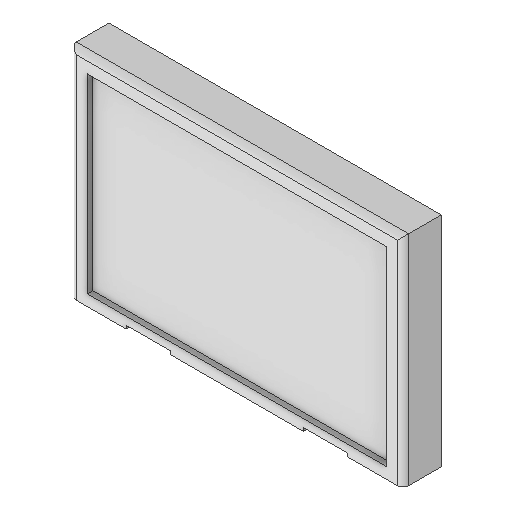
# Autodesk Inventor part: PLATE 2
Saved by Autodesk Inventor 2025.3 (Build 293356030, 356C)
## iProperties
Created: 2025-09-26
Part Number: PLATE 2
Material: 일반
Document SubType Name: Modeling
Designer: joseph
Density: 1 g/cm^3
Appearance: 기본값
Author: joseph
Autodesk Inventor part; units mm, degrees
ref_plane "YZ Plane" through (0, 0, 0) normal (1, 0, 0) x (0, 1, 0)
ref_plane "XZ Plane" through (0, 0, 0) normal (0, 1, 0) x (-1, 0, 0)
ref_plane "XY Plane" through (0, 0, 0) normal (0, 0, 1) x (1, 0, 0)
sketch "스케치1" plane through (0, 0, 0) normal (0, 0, 1) x (1, 0, 0)
  line L0 (150, 3) -> (-150, 3)
  line L1 (-150, 3) -> (-150, 200)
  line L2 (-150, 200) -> (150, 200)
  line L3 (150, 200) -> (150, 3)
  point P0 (0, 0)
  dimension "d0" = 300
  dimension "d1" = 197
  constraints: 8 end point, 2 parallel, 1 horizontal, 1 perpendicular
  measures "d0" distance of L1.end L2.end
  measures "d1" distance of L0.end L1.end
extrude "돌출1" add sketch "스케치1" along normal blind 34.5
fillet "모깎기1" radius 5 3 edges at (150, 101.5, 34.5) (-150, 101.5, 34.5) (0, 200, 34.5)
sketch "스케치2" plane through (0, 0, 0) normal (0, 0, -1) x (-1, 0, 0)
  line L0 (-150, 200) -> (150, 200) projected
  line L1 (-150, 3) -> (-150, 200) projected
  line L2 (150, 3) -> (-150, 3) projected
  line L3 (150, 200) -> (150, 3) projected
  line L4 (-147, 6) -> (-147, 197)
  line L5 (-147, 197) -> (147, 197)
  line L6 (147, 197) -> (147, 6)
  line L7 (147, 6) -> (-147, 6)
  point P0 (0, 0)
  dimension "d5" = 3
  constraints: 8 end point, 3 other
  measures "d5" distance between parallel lines of L2 L7
extrude "돌출2" cut sketch "스케치2" against normal blind 27 contours L4 L5 L6 L7
sketch "스케치3" plane through (-150, 3, 0) normal (-1, 0, 0) x (0, 0, 1)
  line L0 (29.5, 197) -> (29.5, 0) projected
  line L1 (0, 197) -> (29.5, 197) projected
  line L2 (0, 197) -> (0, 0) projected
  line L3 (0, 0) -> (29.5, 0) projected
  line L4 (9.75, 5) -> (19.75, 5)
  line L5 (19.75, 5) -> (19.75, 10)
  line L6 (19.75, 10) -> (9.75, 10)
  line L7 (9.75, 10) -> (9.75, 5)
  point P0 (0, -3)
  point P1 (14.75, 5)
  point P2 (14.75, 0)
  dimension "d8" = 10
  dimension "d9" = 5
  dimension "d10" = 5
  constraints: 8 end point, 2 midpoint, 2 parallel, 1 horizontal, 1 perpendicular, 1 vertical alignment
  measures "d8" distance of L6.end L5.end
  measures "d9" distance of L5.end L4.end
  measures "d10" distance between parallel lines of L3 L4
extrude "돌출3" cut sketch "스케치3" against normal blind 27 contours L7 L6 L5 L4
sketch "스케치4" plane through (0, 0, 34.5) normal (0, 0, 1) x (1, 0, 0)
  line L0 (145, 195) -> (145, 3) projected
  line L1 (-145, 195) -> (145, 195) projected
  line L2 (-145, 3) -> (-145, 195) projected
  line L3 (-145, 3) -> (145, 3) projected
  line L4 (-135, 185) -> (135, 185)
  line L5 (135, 185) -> (135, 13)
  line L6 (135, 13) -> (-135, 13)
  line L7 (-135, 13) -> (-135, 185)
  point P0 (0, 0)
  dimension "d13" = 10
  constraints: 8 end point, 3 other
  measures "d13" distance between parallel lines of L2 L7
extrude "돌출4" cut sketch "스케치4" against normal blind 5 contours L4 L5 L6 L7
sketch "스케치6" plane through (0, 0, 0) normal (0, 0, -1) x (-1, 0, 0)
  line L0 (-147, 197) -> (147, 197) projected
  line L1 (147, 197) -> (147, 6) projected
  line L2 (147, 6) -> (-147, 6) projected
  line L3 (-147, 6) -> (-147, 197) projected
  line L4 (-150, 200) -> (150, 200) projected
  line L5 (-150, 3) -> (-150, 200) projected
  line L6 (150, 3) -> (-150, 3) projected
  line L7 (150, 200) -> (150, 3) projected
  line L8 (-97, 147) -> (97, 147)
  line L9 (97, 147) -> (97, 56)
  line L10 (97, 56) -> (-97, 56)
  line L11 (-97, 56) -> (-97, 147)
  point P0 (0, 0)
  dimension "d16" = 50
  constraints: 8 end point, 3 other
  measures "d16" distance between parallel lines of L3 L11
extrude "돌출5" add sketch "스케치6" against normal blind 3 contours L0 L1 L2 L3
sketch "스케치7" plane through (-150, 3, 0) normal (0, -1, 0) x (1, 0, 0)
  arc A0 (300, 29.5) -> (295, 34.5) centre (295, 29.5) ccw projected
  line L0 (5, 34.5) -> (295, 34.5) projected
  arc A1 (5, 34.5) -> (0, 29.5) centre (5, 29.5) ccw projected
  line L1 (0, 0) -> (0, 29.5) projected
  line L2 (0, 0) -> (300, 0) projected
  line L3 (300, 0) -> (300, 29.5) projected
  line L4 (50, 34.5) -> (90, 34.5)
  line L5 (90, 34.5) -> (90, 18.5)
  line L6 (90, 18.5) -> (50, 18.5)
  line L7 (50, 18.5) -> (50, 34.5)
  line L8 (210, 34.5) -> (250, 34.5)
  line L9 (250, 34.5) -> (250, 18.5)
  line L10 (250, 18.5) -> (210, 18.5)
  line L11 (210, 18.5) -> (210, 34.5)
  point P0 (150, 0)
  dimension "d19" = 40
  dimension "d20" = 16
  dimension "d21" = 40
  dimension "d22" = 16
  dimension "d23" = 50
  dimension "d24" = 50
  constraints: 16 end point, 4 parallel, 2 horizontal, 2 perpendicular, 2 point on line
  measures "d19" distance of L5.end L6.end
  measures "d20" distance of L4.end L5.end
  measures "d21" distance of L9.end L10.end
  measures "d22" distance of L8.end L9.end
  measures "d23" distance from line of L7 L1.start
  measures "d24" distance from line of L3 L9.end
extrude "돌출6" cut sketch "스케치7" against normal blind 1 contours L9 L10 L11 L0 | L5 L6 L7 L0
fillet "모깎기2" radius 2 2 edges at (-80, 4, 34.5) (80, 4, 34.5) inverted yes
sketch "스케치8" plane through (97, 56, 0) normal (-1, 0, 0) x (0, 0, 1)
  line L0 (0, 0) -> (0, 91) projected
  line L1 (0, 0) -> (3, 0) projected
  line L2 (3, 91) -> (3, 0) projected
  line L3 (0, 91) -> (3, 91) projected
  line L4 (0, 86) -> (9, 86)
  line L5 (9, 86) -> (9, 71)
  line L6 (9, 71) -> (0, 71)
  line L7 (0, 71) -> (0, 86)
  line L8 (0, 20) -> (9, 20)
  line L9 (9, 20) -> (9, 5)
  line L10 (9, 5) -> (0, 5)
  line L11 (0, 5) -> (0, 20)
  line L12 (3, 74) -> (6, 74)
  line L13 (6, 74) -> (6, 83)
  line L14 (6, 83) -> (3, 83)
  line L15 (3, 83) -> (3, 74)
  line L16 (6, 8) -> (6, 17)
  line L17 (6, 17) -> (3, 17)
  line L18 (3, 17) -> (3, 8)
  line L19 (3, 8) -> (6, 8)
  point P0 (0, -56)
  point P1 (3, 20)
  point P2 (3, 17)
  point P3 (3, 8)
  point P4 (3, 5)
  point P5 (3, 86)
  point P6 (3, 71)
  dimension "d28" = 9
  dimension "d29" = 15
  dimension "d30" = 15
  dimension "d31" = 5
  dimension "d32" = 5
  dimension "d33" = 3
  dimension "d34" = 3
  constraints: 32 end point, 8 parallel, 4 perpendicular, 3 point on line, 2 horizontal, 6 other
  measures "d28" distance of L5.end L6.end
  measures "d29" distance of L4.end L5.end
  measures "d30" distance of L8.end L9.end
  measures "d31" distance from line of L2.start L4
  measures "d32" distance from line of L0.start L10
  measures "d33" distance between parallel lines of L6 L12
  measures "d34" distance between parallel lines of L9 L16
extrude "돌출7" add sketch "스케치8" against normal blind 10 contours L2 L19 L16 L17 L8 L9 L10 | L2 L12 L13 L14 L4 L5 L6
fillet "모깎기3" radius 2 2 edges at (97, 68.5, 3) (97, 134.5, 3)
sketch "스케치9" plane through (0, 0, 3) normal (0, 0, 1) x (1, 0, 0)
  line L0 (147, 6) -> (-147, 6) projected
  line L1 (147, 197) -> (147, 6) projected
  line L2 (-147, 197) -> (147, 197) projected
  line L3 (-147, 6) -> (-147, 197) projected
  line L4 (97, 76) -> (107, 76) projected
  line L5 (107, 76) -> (107, 73) projected
  line L6 (107, 73) -> (99, 73) projected
  line L7 (99, 64) -> (107, 64) projected
  line L8 (107, 64) -> (107, 61) projected
  line L9 (107, 61) -> (97, 61) projected
  line L10 (97, 61) -> (97, 56) projected
  line L11 (97, 56) -> (-97, 56) projected
  line L12 (-97, 56) -> (-97, 147) projected
  line L13 (-97, 147) -> (97, 147) projected
  line L14 (97, 147) -> (97, 142) projected
  line L15 (97, 142) -> (107, 142) projected
  line L16 (107, 142) -> (107, 139) projected
  line L17 (107, 139) -> (99, 139) projected
  line L18 (99, 130) -> (107, 130) projected
  line L19 (107, 130) -> (107, 127) projected
  line L20 (107, 127) -> (97, 127) projected
  line L21 (97, 127) -> (97, 76) projected
  line L22 (-112, 121.5) -> (-97, 121.5)
  line L23 (-97, 121.5) -> (-97, 81.5)
  line L24 (-97, 81.5) -> (-112, 81.5)
  line L25 (-112, 81.5) -> (-112, 121.5)
  line L26 (99, 130) -> (99, 139) projected
  line L27 (99, 64) -> (99, 73) projected
  point P0 (0, 0)
  point P1 (-97, 101.5)
  dimension "d38" = 15
  dimension "d39" = 40
  constraints: 8 end point, 2 midpoint, 2 parallel, 1 horizontal, 1 perpendicular
  measures "d38" distance of L23.end L24.end
  measures "d39" distance of L22.end L23.end
extrude "돌출8" add sketch "스케치9" along normal blind 3 contours L24 L25 L22 L12
sketch "스케치10" plane through (0, 0, 0) normal (0, 0, -1) x (-1, 0, 0)
  line L0 (-97, 147) -> (97, 147) projected
  line L1 (97, 147) -> (97, 56) projected
  line L2 (97, 56) -> (-97, 56) projected
  line L3 (-97, 56) -> (-97, 147) projected
  line L4 (-150, 200) -> (150, 200) projected
  line L5 (-150, 3) -> (-150, 200) projected
  line L6 (150, 3) -> (-150, 3) projected
  line L7 (150, 200) -> (150, 3) projected
  line L8 (110, 86.5) -> (97, 86.5)
  line L9 (97, 86.5) -> (97, 116.5)
  line L10 (97, 116.5) -> (110, 116.5)
  line L11 (110, 116.5) -> (110, 86.5)
  point P0 (0, 0)
  point P1 (97, 101.5)
  dimension "d42" = 13
  dimension "d43" = 30
  constraints: 8 end point, 2 midpoint, 2 parallel, 1 horizontal, 1 perpendicular
  measures "d42" distance of L9.end L10.end
  measures "d43" distance of L8.end L9.end
extrude "돌출9" cut sketch "스케치10" against normal blind 3 contours L10 L11 L8 L1
sketch "스케치11" plane through (0, 0, 3) normal (0, 0, -1) x (-1, 0, 0)
  line L0 (97, 116.5) -> (110, 116.5) projected
  line L1 (97, 86.5) -> (97, 116.5) projected
  line L2 (110, 86.5) -> (97, 86.5) projected
  line L3 (110, 116.5) -> (110, 86.5) projected
  circle A0 centre (103.5, 94.5) radius 1.5
  circle A1 centre (103.5, 108.5) radius 1.5
  point P0 (0, 0)
  dimension "d46" = 3
  dimension "d47" = 3
  dimension "d48" = 8
  dimension "d49" = 8
  constraints: 2 centre point
  measures "d46" diameter of A0
  measures "d47" diameter of A1
  measures "d48" distance from line of L2 A0.centre
  measures "d49" distance from line of L0 A1.centre
extrude "돌출10" cut sketch "스케치11" against normal blind 10 contours A0 | A1
sketch "스케치12" plane through (0, 0, 6) normal (0, 0, 1) x (1, 0, 0)
  circle A0 centre (-103.5, 108.5) radius 1.5 projected
  circle A1 centre (-103.5, 94.5) radius 1.5 projected
  line L0 (-112, 81.5) -> (-97, 81.5) projected
  line L1 (-97, 81.5) -> (-97, 121.5) projected
  line L2 (-97, 121.5) -> (-112, 121.5) projected
  line L3 (-112, 121.5) -> (-112, 81.5) projected
  line L4 (-101.8834, 105.7) -> (-105.1166, 105.7)
  line L5 (-105.1166, 105.7) -> (-106.7332, 108.5)
  line L6 (-106.7332, 108.5) -> (-105.1166, 111.3)
  line L7 (-105.1166, 111.3) -> (-101.8834, 111.3)
  line L8 (-101.8834, 111.3) -> (-100.2668, 108.5)
  line L9 (-100.2668, 108.5) -> (-101.8834, 105.7)
  line L10 (-100.7287, 113.3) -> (-106.2713, 113.3)
  line L11 (-106.2713, 113.3) -> (-109.0426, 108.5)
  line L12 (-109.0426, 108.5) -> (-106.2713, 103.7)
  line L13 (-106.2713, 103.7) -> (-100.7287, 103.7)
  line L14 (-100.7287, 103.7) -> (-97.9574, 108.5)
  line L15 (-97.9574, 108.5) -> (-100.7287, 113.3)
  circle A2 centre (-103.5, 94.5) radius 1.5
  line L16 (-101.8834, 91.7) -> (-105.1166, 91.7)
  line L17 (-105.1166, 91.7) -> (-106.7332, 94.5)
  line L18 (-106.7332, 94.5) -> (-105.1166, 97.3)
  line L19 (-105.1166, 97.3) -> (-101.8834, 97.3)
  line L20 (-101.8834, 97.3) -> (-100.2668, 94.5)
  line L21 (-100.2668, 94.5) -> (-101.8834, 91.7)
  line L22 (-100.7287, 99.3) -> (-106.2713, 99.3)
  line L23 (-106.2713, 99.3) -> (-109.0426, 94.5)
  line L24 (-109.0426, 94.5) -> (-106.2713, 89.7)
  line L25 (-106.2713, 89.7) -> (-100.7287, 89.7)
  line L26 (-100.7287, 89.7) -> (-97.9574, 94.5)
  line L27 (-97.9574, 94.5) -> (-100.7287, 99.3)
  point P0 (0, 0)
  dimension "d52" = 5.6
  dimension "d53" = 2
  dimension "d54" = 5.6
  dimension "d55" = 2
  constraints: 48 end point, 2 coincident, 2 horizontal, 1 centre point, 36 other
  measures "d52" distance between parallel lines of L9 L6
  measures "d53" distance between parallel lines of L7 L10
  measures "d54" distance between parallel lines of L21 L18
  measures "d55" distance between parallel lines of L19 L22
extrude "돌출11" add sketch "스케치12" along normal blind 3 contours L15 L14 L13 L12 L11 L10 | L27 L26 L25 L24 L23 L22
